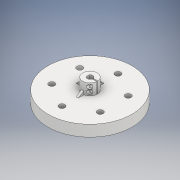
# Autodesk Inventor part: MC001
Saved by Autodesk Inventor 2017 SP1 (Build 210196100, 196)
## iProperties
Created: 2017-06-01
Part Number: MC001
Material: ABS Plastic
Document SubType Name: Modeling
Designer: Zach
Density: 1.06 g/cm^3
Appearance: CR White
Author: Zach
Autodesk Inventor part; units mm, degrees
ref_plane "YZ Plane" through (0, 0, 0) normal (1, 0, 0) x (0, 1, 0)
ref_plane "XY Plane" through (0, 0, 0) normal (0, 0, 1) x (1, 0, 0)
sketch "Sketch1" plane through (0, 0, 0) normal (0, 0, 1) x (1, 0, 0)
  circle A0 centre (0, 0) radius 37.5
  circle A1 centre (0, 0) radius 2.5
  circle A2 centre (0, 25) radius 2.575
  circle A3 centre (-21.6506, 12.5) radius 2.575
  circle A4 centre (-21.6506, -12.5) radius 2.575
  circle A5 centre (0, -25) radius 2.575
  circle A6 centre (21.6506, -12.5) radius 2.575
  circle A7 centre (21.6506, 12.5) radius 2.575
  dimension "d0" = 75
  dimension "d1" = 5
  dimension "d2" = 5.15
  dimension "d3" = 25
  dimension "d6" = 360
  constraints: 8 centre point, 2 coincident, 13 other
  measures "d0" diameter of A0
  measures "d1" diameter of A1
  measures "d2" diameter of A2
  measures "d3" distance of point (0, 0) A2.centre
extrude "Extrusion1" add sketch "Sketch1" along normal blind 10
sketch "Sketch2" plane through (0, 0, 10) normal (0, 0, 1) x (1, 0, 0)
  circle A0 centre (0, 0) radius 2.5 projected
  circle A1 centre (0, 0) radius 6.5
  circle A2 centre (0, 0) radius 2.5 projected
  dimension "d10" = 13
  constraints: 3 coincident, 1 centre point, 3 other
  measures "d10" diameter of A1
extrude "Extrusion2" add sketch "Sketch2" along normal blind 10
sketch "Sketch3" plane through (0, 0, 10) normal (0, 0, 1) x (1, 0, 0)
  line L0 (0, 0.5) -> (37.4967, 0.5)
  circle A0 centre (0, 0) radius 6.5 projected
  line L1 (0, 0.5) -> (0, -0.5)
  circle A1 centre (0, 0) radius 37.5 projected
  line L2 (0, -0.5) -> (37.4967, -0.5)
  arc A2 (37.4967, -0.5) -> (37.4967, 0.5) centre (0, 0) ccw
  point P0 (0, 0)
  dimension "d13" = 1
  dimension "d14" = 0.5
  constraints: 6 end point, 4 point on circle, 2 horizontal, 2 vertical alignment, 1 centre point, 1 concentric, 1 midpoint, 1 vertical
  measures "d13" distance of L0.start L1.end
  measures "d14" distance of L0.start point (0, 0)
extrude "Extrusion4" cut sketch "Sketch3" along normal through all contours L0 A0 L2 L1 | L0 A1 L2 A0 picked at (2.1667, 0) picked at (16.8315, -0.2223)
sketch "Sketch4" plane through (0, 0, 0) normal (0, 1, 0) x (-1, 0, 0)
  circle A0 centre (-4.4495, 13) radius 1
  circle A1 centre (-4.4495, 17) radius 1
  line L0 (-2.4495, 10) -> (-6.4807, 10) projected
  line L1 (-6.4807, 20) -> (-2.4495, 20) projected
  line L2 (-2.4495, 20) -> (-2.4495, 10) projected
  point P0 (0, 0)
  dimension "d19" = 2
  dimension "d20" = 2
  dimension "d21" = 3
  dimension "d22" = 3
  dimension "d25" = 2
  dimension "d26" = 2
  constraints: 2 centre point
  measures "d19" diameter of A0
  measures "d20" diameter of A1
  measures "d21" distance from line of A0.centre L0
  measures "d22" distance from line of L1 A1.centre
  measures "d25" distance from line of L2 A0.centre
  measures "d26" distance from line of L2 A1.centre
extrude "Extrusion5" cut sketch "Sketch4" along normal through all both and the other way through all
ref_plane "Work Plane1" through (0, -6.5, 0) normal (0, 1, 0) x (-1, 0, 0)
sketch "Sketch6" plane through (0, -6.5, 0) normal (0, 1, 0) x (-1, 0, 0)
  spline S0 degree 5 poles (-3.4495, 13) (-3.4495, 13.1717) (-3.486, 13.3437) (-3.5604, 13.5053) (-3.6677, 13.6465) (-3.897, 13.8439) (-4.0102, 13.9123) (-4.1302, 13.9602) (-4.2518, 13.9875) (-4.571, 14.0127) (-4.7636, 13.9773) (-4.9359, 13.9015) (-5.0869, 13.7934) (-5.2938, 13.5513) (-5.3641, 13.4364) (-5.4202, 13.3045) (-5.4495, 13.152) (-5.4495, 12.8771) (-5.4304, 12.7538) (-5.3933, 12.6417) (-5.3442, 12.5407) (-5.2314, 12.3689) (-5.1691, 12.296) (-5.1, 12.232) (-5.025, 12.177) (-4.8442, 12.074) (-4.7351, 12.031) (-4.6186, 12.0034) (-4.4963, 11.9932) (-4.2525, 12.0124) (-4.1316, 12.0395) (-4.0123, 12.0868) (-3.8997, 12.1545) (-3.6697, 12.3509) (-3.5614, 12.4925) (-3.4863, 12.6547) (-3.4495, 12.8276) (-3.4495, 13) knots 0 0 0 0 0 0 0.126407 0.126407 0.126407 0.126407 0.224001 0.224001 0.224001 0.224001 0.387733 0.387733 0.387733 0.387733 0.499705 0.499705 0.499705 0.499705 0.590268 0.590268 0.590268 0.590268 0.67301 0.67301 0.67301 0.67301 0.775734 0.775734 0.775734 0.775734 0.872864 0.872864 0.872864 0.872864 1 1 1 1 1 1 projected
  spline S1 degree 5 poles (-3.4495, 17) (-3.4495, 17.1717) (-3.486, 17.3437) (-3.5604, 17.5053) (-3.6677, 17.6465) (-3.897, 17.8439) (-4.0102, 17.9123) (-4.1302, 17.9602) (-4.2518, 17.9875) (-4.571, 18.0127) (-4.7636, 17.9773) (-4.9359, 17.9015) (-5.0869, 17.7934) (-5.2938, 17.5513) (-5.3641, 17.4364) (-5.4202, 17.3045) (-5.4495, 17.152) (-5.4495, 16.8771) (-5.4304, 16.7538) (-5.3933, 16.6417) (-5.3442, 16.5407) (-5.2314, 16.3689) (-5.1691, 16.296) (-5.1, 16.232) (-5.025, 16.177) (-4.8442, 16.074) (-4.7351, 16.031) (-4.6186, 16.0034) (-4.4963, 15.9932) (-4.2525, 16.0124) (-4.1316, 16.0395) (-4.0123, 16.0868) (-3.8997, 16.1545) (-3.6697, 16.3509) (-3.5614, 16.4925) (-3.4863, 16.6547) (-3.4495, 16.8276) (-3.4495, 17) knots 0 0 0 0 0 0 0.126407 0.126407 0.126407 0.126407 0.224001 0.224001 0.224001 0.224001 0.387733 0.387733 0.387733 0.387733 0.499705 0.499705 0.499705 0.499705 0.590268 0.590268 0.590268 0.590268 0.67301 0.67301 0.67301 0.67301 0.775734 0.775734 0.775734 0.775734 0.872864 0.872864 0.872864 0.872864 1 1 1 1 1 1 projected
  circle A0 centre (-4.4495, 13) radius 1 projected
  circle A1 centre (-4.4495, 17) radius 1 projected
  line L0 (-5.4495, 11.2679) -> (-6.4495, 13)
  line L1 (-6.4495, 13) -> (-5.4495, 14.7321)
  line L2 (-5.4495, 14.7321) -> (-3.4495, 14.7321)
  line L3 (-3.4495, 14.7321) -> (-2.4495, 13)
  line L4 (-2.4495, 13) -> (-3.4495, 11.2679)
  line L5 (-3.4495, 11.2679) -> (-5.4495, 11.2679)
  line L6 (-5.4495, 15.2679) -> (-6.4495, 17)
  line L7 (-6.4495, 17) -> (-5.4495, 18.7321)
  line L8 (-5.4495, 18.7321) -> (-3.4495, 18.7321)
  line L9 (-3.4495, 18.7321) -> (-2.4495, 17)
  line L10 (-2.4495, 17) -> (-3.4495, 15.2679)
  line L11 (-3.4495, 15.2679) -> (-5.4495, 15.2679)
  point P0 (0, 0)
  dimension "d30" = 2
  dimension "d31" = 2
  constraints: 24 end point, 4 horizontal alignment, 2 coincident, 28 other
  measures "d30" distance of L6.end point (-4.449, 17)
  measures "d31" distance of L0.end point (-4.449, 13)
extrude "Extrusion6" cut sketch "Sketch6" along normal blind 3
sketch "Sketch7" plane through (0, 0, 0) normal (1, 0, 0) x (0, 1, 0)
  line L0 (6.5, 13) -> (11.5, 10)
  line L1 (37.5, 10) -> (-37.5, 10) projected
  line L2 (-6.5, 10) -> (6.5, 10) projected
  line L3 (6.5, 10) -> (11.5, 10)
  line L4 (6.5, 10) -> (5.5, 10)
  line L5 (5.5, 10) -> (5.5, 13)
  line L6 (5.5, 13) -> (6.5, 13)
  line L7 (6.5, 10) -> (6.5, 20) projected
  line L8 (0, 0) -> (0, 35.1607) construction
  line L9 (-6.5, 13) -> (-11.5, 10)
  line L10 (-37.5, 10) -> (37.5, 10)
  line L11 (6.5, 10) -> (-6.5, 10)
  line L12 (-6.5, 10) -> (-11.5, 10)
  line L13 (-6.5, 10) -> (-5.5, 10)
  line L14 (-5.5, 10) -> (-5.5, 13)
  line L15 (-5.5, 13) -> (-6.5, 13)
  point P0 (-0.5, 10)
  point P1 (0.5, 10)
  dimension "d36" = 5
  dimension "d39" = 3
  dimension "d46" = 1
  dimension "d53" = 5
  constraints: 26 end point, 7 symmetric about line, 5 point on line, 2 vertical, 1 perpendicular, 2 other
  measures "d36" horizontal distance of L0.start L0.end
  measures "d39" vertical distance of L0.start L0.end
  measures "d46" distance of L2.end L4.end
  measures "d53" horizontal distance of L9.start L9.end
extrude "Extrusion7" add sketch "Sketch7" along normal mid plane 2
sketch "Sketch8" plane through (0, 0, 0) normal (0, 1, 0) x (-1, 0, 0)
  line L0 (6.5, 13) -> (11.5, 10)
  line L1 (37.5, 10) -> (-37.5, 10) projected
  line L2 (0.5095, 10) -> (0.5095, 16.5943)
  line L3 (11.5, 10) -> (0.5095, 10)
  line L4 (6.5, 13) -> (5.5, 13)
  line L5 (6.5, 10) -> (6.5, 20) projected
  line L6 (6.5, 13) -> (7.5, 13) construction
  line L7 (5.5, 13) -> (5.5, 10)
  line L8 (1, 10) -> (6.5, 10) projected
  line L9 (6.5, 10) -> (5.5, 10)
  point P0 (0, 0)
  dimension "d42" = 5
  dimension "d43" = 3
  dimension "d51" = 1
  dimension "d52" = 180
  constraints: 14 end point, 4 point on line, 2 collinear, 2 perpendicular, 2 vertical, 1 horizontal
  measures "d42" horizontal distance of L0.start L0.end
  measures "d43" vertical distance of L0.start L0.end
  measures "d51" distance of L0.start L4.end
  measures "d52" angle of L4 L6
extrude "Extrusion8" add sketch "Sketch8" along normal mid plane 2
sketch "Sketch9" plane through (0, 0, 0) normal (0, 0, -1) x (-1, 0, 0)
  circle A0 centre (0, 0) radius 2.5 projected
  line L0 (2, -1.5) -> (2, 1.5)
  arc A1 (2, -1.5) -> (2, 1.5) centre (0, 0) ccw
  dimension "d54" = 2
  constraints: 4 point on circle, 2 end point, 1 centre point, 1 concentric, 1 vertical
  measures "d54" distance from line of point (0, 0) L0
extrude "Extrusion9" add sketch "Sketch9" against normal blind 20 contours A0 L0 picked at (2.0912, -0.3466)
body "Solid1"
